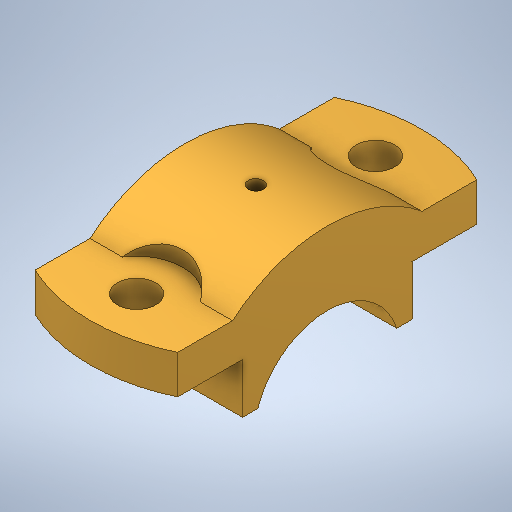
# Autodesk Inventor part: cap
Saved by Autodesk Inventor 2025.2 (Build 292293000, 293)
## iProperties
Created: 2025-04-15
Part Number: cap
Material: Brass, Soft Yellow
Document SubType Name: Modeling
Designer: bless
Density: 8.47 g/cm^3
Appearance: Brass - Satin
Author: bless
Autodesk Inventor part; units mm, degrees
ref_plane "YZ Plane" through (0, 0, 0) normal (1, 0, 0) x (0, 1, 0)
ref_plane "XZ Plane" through (0, 0, 0) normal (0, 1, 0) x (-1, 0, 0)
ref_plane "XY Plane" through (0, 0, 0) normal (0, 0, 1) x (1, 0, 0)
sketch "Sketch1" plane through (0, 0, 0) normal (0, 1, 0) x (-1, 0, 0)
  circle A0 centre (0, 0) radius 2
  line L0 (-18.4961, 38.8165) -> (-18.4961, -38.8135)
  line L1 (18.4961, 38.8135) -> (-18.4961, -38.8135) construction
  line L2 (-18.4961, 38.8165) -> (18.4961, -38.8165) construction
  circle A1 centre (0, 31) radius 5
  circle A2 centre (0, -31) radius 5
  arc A3 (18.5039, 38.815) -> (-18.4961, 38.8188) centre (0, 0) ccw
  arc A4 (-18.4961, -38.8188) -> (18.5039, -38.815) centre (0, 0) ccw
  line L3 (18.5039, 38.815) -> (18.5039, -38.815)
  line L4 (-18.4961, -38.8135) -> (-18.4961, -38.8188)
  line L5 (-18.4961, 38.8165) -> (-18.4961, 38.8188)
  dimension "d0" = 2
  dimension "d4" = 10
  dimension "d5" = 10
  dimension "d6" = 31
  dimension "d7" = 31
  dimension "d8" = 77.63
  dimension "d9" = 37
  dimension "d10" = 43
  dimension "d11" = 43
  dimension "d12" = 77.63
  constraints: 12 end point, 5 centre point, 4 point on circle, 2 coincident, 2 midpoint, 2 parallel, 2 point on line, 2 vertical alignment
  measures "d0" radius of A0
  measures "d4" diameter of A1
  measures "d5" diameter of A2
  measures "d6" distance of A1.centre point (0, 0)
  measures "d7" distance of A2.centre point (0, 0)
  measures "d8" distance of L0.start L0.end
  measures "d9" distance between parallel lines of L0 L3
  measures "d10" radius of A4
  measures "d11" radius of A3
  measures "d12" distance of L3.start L3.end
extrude "Extrusion1" add sketch "Sketch1" along normal blind 10
sketch "Sketch2" plane through (18.4961, 0, 38.8188) normal (1, 0, 0) x (0, 0, -1)
  line L0 (0, 0) -> (77.6375, 0) projected
  line L1 (0, 10) -> (77.6375, 10) projected
  line L2 (0.0038, 0) -> (-4.1812, 0) projected
  line L3 (-4.1812, 0) -> (16.8188, 0)
  line L4 (16.8188, 0) -> (16.8188, -13)
  line L5 (16.8188, -13) -> (20.7888, -13)
  line L6 (81.8188, 0) -> (77.6338, 0) projected
  line L7 (81.8188, 0) -> (60.8188, 0)
  line L8 (60.8188, 0) -> (60.8188, -13)
  line L9 (60.8188, -13) -> (56.8488, -13)
  arc A0 (56.8488, -13) -> (20.7888, -13) centre (38.8188, -19.0031) ccw
  arc A1 (63.4021, 10) -> (14.2354, 10) centre (38.8188, -19.0031) ccw
  line L10 (36.8188, 10) -> (40.8188, 10) projected
  point P0 (38.8188, 0)
  point P1 (38.8188, 19.0169)
  dimension "d15" = 21
  dimension "d16" = 13
  dimension "d17" = 3.97
  dimension "d18" = 21
  dimension "d19" = 13
  dimension "d20" = 3.97
  dimension "d22" = 38.02
  constraints: 12 end point, 6 point on circle, 4 perpendicular, 4 point on line, 2 centre point, 1 concentric, 1 vertical alignment
  measures "d15" distance of L2.end L3.end
  measures "d16" distance of L3.end L4.end
  measures "d17" distance of L4.end L5.end
  measures "d18" distance of L6.start L7.end
  measures "d19" distance of L7.end L8.end
  measures "d20" distance of L8.end L9.end
  measures "d22" radius of A1
extrude "Extrusion2" add sketch "Sketch2" against normal blind 37
sketch "Sketch3" plane through (0, 10, 0) normal (0, -1, 0) x (1, 0, 0)
  circle A0 centre (0, 0) radius 2 projected
extrude "Extrusion3" cut sketch "Sketch3" along normal through all both and the other way through all
sketch "Sketch4" plane through (0, 0, 0) normal (0, -1, 0) x (1, 0, 0)
  circle A0 centre (0, 31) radius 5 projected
  arc A1 (-12, 31) -> (12, 31) centre (0, 31) ccw
  circle A2 centre (0, 31) radius 10.5 projected
  arc A3 (-10.5, 31) -> (10.5, 31) centre (0, 31) ccw
  line L0 (12, 31) -> (-12, 31)
  point P0 (10.5, 31)
  dimension "d27" = 12
  constraints: 4 point on circle, 2 centre point, 2 coincident, 2 end point, 2 point on line, 1 concentric, 1 midpoint
  measures "d27" radius of A1
extrude "Extrusion4" cut sketch "Sketch4" against normal blind 3.032 from surface at -10 contours L0 A1 A2
sketch "Sketch5" plane through (0, 10, 0) normal (0, 1, 0) x (1, 0, 0)
  line L0 (-18.5039, 24.5833) -> (18.4961, 24.5833) projected
  circle A0 centre (0, 31) radius 5 projected
  circle A1 centre (0, 31) radius 10.5 projected
  arc A2 (-12, 31) -> (12, 31) centre (0, 31) ccw
  arc A3 (-10.5, 31) -> (10.5, 31) centre (0, 31) ccw
  line L1 (12, 31) -> (-12, 31)
  point P0 (8.3112, 24.5833)
  point P1 (-8.3112, 24.5833)
  dimension "d30" = 12
  constraints: 4 point on circle, 2 centre point, 2 coincident, 2 end point, 2 point on line, 1 concentric, 1 horizontal, 1 midpoint
  measures "d30" radius of A2
extrude "Extrusion5" cut sketch "Sketch5" along normal through all contours A2 L1 A1 L0 | L0 A1 A2 | L0 A1 | L0 A1 L1 A2
sketch "Sketch6" plane through (0, 13.032, 31) normal (0, -1, 0) x (1, 0, 0)
  arc A0 (-5.7661, -10.5239) -> (5.7661, -10.5239) centre (0, 0) ccw projected
  line L0 (-5.7661, -10.5239) -> (5.7661, -10.5239) projected
  spline S0 degree 6 poles (8.3112, -6.4167) (8.1303, -6.651) (7.9395, -6.8817) (7.739, -7.108) (7.5289, -7.3291) (7.3096, -7.5442) (6.6527, -8.1442) (6.1935, -8.5115) (5.7064, -8.85) (5.1948, -9.156) (4.663, -9.4266) (3.9079, -9.7483) (3.6976, -9.8316) (3.4851, -9.9094) (3.2708, -9.9817) (3.0547, -10.0484) (2.3754, -10.239) (1.9069, -10.3432) (1.4335, -10.4215) (0.9567, -10.4739) (0.4783, -10.5) (-0.4841, -10.5) (-0.9683, -10.4732) (-1.4508, -10.4196) (-1.9299, -10.3394) (-2.4038, -10.2327) (-3.0854, -10.0389) (-3.2986, -9.9724) (-3.5101, -9.9004) (-3.7198, -9.8231) (-3.9273, -9.7404) (-4.6765, -9.4197) (-5.2053, -9.1498) (-5.7139, -8.8448) (-6.1983, -8.5077) (-6.655, -8.1422) (-7.3097, -7.5441) (-7.529, -7.3291) (-7.739, -7.108) (-7.9396, -6.8817) (-8.1303, -6.6509) (-8.3112, -6.4167) knots 0 0 0 0 0 0 0 0.097765 0.097765 0.097765 0.097765 0.097765 0.281656 0.281656 0.281656 0.281656 0.281656 0.351588 0.351588 0.351588 0.351588 0.351588 0.499999 0.499999 0.499999 0.499999 0.499999 0.65021 0.65021 0.65021 0.65021 0.65021 0.719277 0.719277 0.719277 0.719277 0.719277 0.902242 0.902242 0.902242 0.902242 0.902242 1 1 1 1 1 1 1 projected
  line L1 (8.3112, -6.4167) -> (-8.3112, -6.4167) projected
  point P0 (0, -31)
  constraints: 1 horizontal alignment
extrude "Extrusion6" cut sketch "Sketch6" against normal blind 10 from surface at 3.032
body "Solid1"
